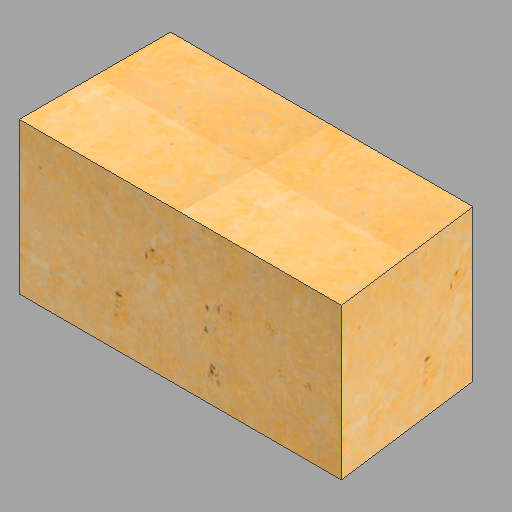
# Autodesk Inventor part: A - 1
Saved by Autodesk Inventor 2023 (Build 270158000, 158)
## iProperties
RuleStatus: InUse
Created: 2022-04-25
Part Number: A - 1
Material: Granite, Cut, Polished
Document SubType Name: Modeling
Designer: awelt
Mass: 1.26311e+06 g
Surface Area: 38160.3 cm^2
Volume: 467818 cm^3
Density: 2.7 g/cm^3
Appearance: Amber Select
AfterDocSave0: Convert in3 volume to ft3
in3 to ft3: 16.52
TEST: 16.521
Author: awelt
Autodesk Inventor part; units mm, degrees
ref_plane "YZ Plane" through (0, 0, 0) normal (1, 0, 0) x (0, 1, 0)
ref_plane "XZ Plane" through (0, 0, 0) normal (0, 1, 0) x (-1, 0, 0)
ref_plane "XY Plane" through (0, 0, 0) normal (0, 0, 1) x (1, 0, 0)
sketch "Sketch1" plane through (0, 0, 0) normal (0, 1, 0) x (-1, 0, 0)
  line L0 (0, 0) -> (-1219.2, 0)
  line L1 (0, 0) -> (0, 609.6)
  line L2 (0, 609.6) -> (-1298.575, 609.6)
  line L3 (-1298.575, 609.6) -> (-1219.2, 0)
  dimension "d0" = 1219.2
  dimension "d1" = 1298.575
  dimension "d2" = 609.6
  constraints: 8 end point, 2 horizontal, 1 vertical
  measures "d0" distance of L0.start L0.end
  measures "d1" distance of L1.end L2.end
  measures "d2" distance of L0.start L1.end
extrude "Extrusion1" add sketch "Sketch1" along normal blind 609.6
body "Solid1"
